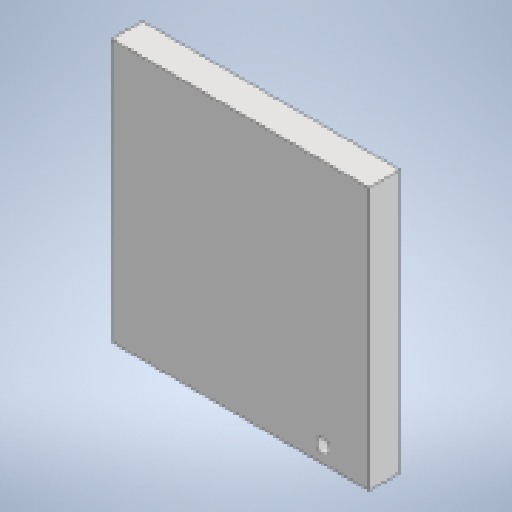
# Autodesk Inventor part: head_side
Saved by Autodesk Inventor 2024 (Build 280153000, 153)
## iProperties
Created: 2024-09-18
Part Number: head_side
Material: 일반
Document SubType Name: Modeling
Designer: Eungang
Density: 1 g/cm^3
Appearance: 기본값
Author: Eungang
Autodesk Inventor part; units mm, degrees
ref_plane "YZ Plane" through (0, 0, 0) normal (1, 0, 0) x (0, 1, 0)
ref_plane "XZ Plane" through (0, 0, 0) normal (0, 1, 0) x (-1, 0, 0)
ref_plane "XY Plane" through (0, 0, 0) normal (0, 0, 1) x (1, 0, 0)
sketch "스케치1" plane through (0, 0, 0) normal (0, 0, 1) x (1, 0, 0)
  line L0 (0, 0) -> (50, 0) projected
  line L1 (50, 0) -> (50, 25) projected
  line L2 (0, 25) -> (50, 25) projected
  line L3 (0, 0) -> (0, 25) projected
  line L4 (8.4, 0) -> (0, 0) projected
  line L5 (0, 0) -> (0, -16) projected
  line L6 (50, -16) -> (0, -16) projected
  line L7 (50, 0) -> (50, -16) projected
  line L8 (50, 0) -> (41.6, 0) projected
  line L9 (41.6, 0) -> (41.6, -10) projected
  line L10 (41.6, -10) -> (8.4, -10) projected
  line L11 (8.4, 0) -> (8.4, -10) projected
  line L12 (0, 25) -> (50, 25)
  line L13 (50, 25) -> (50, 35)
  line L14 (50, 35) -> (0, 35)
  line L15 (0, 35) -> (0, 25)
  line L16 (0, -16) -> (50, -16)
  line L17 (50, -16) -> (50, 35)
  line L18 (50, 35) -> (0, 35)
  line L19 (0, 35) -> (0, -16)
  dimension "d0" = 10
  constraints: 16 end point, 4 parallel, 2 horizontal, 2 perpendicular, 1 point on line
  measures "d0" distance of L13.end L12.end
extrude "돌출1" add sketch "스케치1" along normal blind 6
sketch "스케치2" plane through (0, 0, 6) normal (0, 0, 1) x (1, 0, 0)
  circle A0 centre (41, -13) radius 1.35 projected
  point P0 (0, 0)
extrude "돌출2" cut sketch "스케치2" against normal up to next
sketch "스케치3" plane through (0, 35, 0) normal (0, 1, 0) x (1, 0, 0)
  line L0 (50, 0) -> (0, 0) projected
  line L1 (28, -6) -> (50, -6) projected
  line L2 (39, -6) -> (25, 0)
  line L3 (39, -6) -> (22, -6)
  line L4 (22, -6) -> (22, 0)
  line L5 (22, 0) -> (39, 0)
  line L6 (39, 0) -> (39, -6)
  line L7 (39, 0) -> (28, 0)
  line L8 (28, 0) -> (28, -6)
  line L9 (28, -6) -> (39, -6)
  line L10 (39, -6) -> (39, 0)
  point P0 (22, -6)
  constraints: 18 end point, 4 parallel, 2 horizontal, 2 midpoint, 2 perpendicular, 2 point on line
extrude "돌출3" add sketch "스케치3" along normal blind 6 contours L8 L2 L0 | L2 L8 L3 L4 L0
sketch "스케치4" plane through (50, 35, 6) normal (0, 1, 0) x (1, 0, 0)
  circle A0 centre (-4.2, 79) radius 1.35 projected
  circle A1 centre (-4.2, 3) radius 1.35 projected
  circle A2 centre (-45.8, 79) radius 1.35 projected
  circle A3 centre (-45.8, 3) radius 1.35 projected
  circle A4 centre (-4.2, 71.8) radius 1.6 projected
  circle A5 centre (-45.8, 71.8) radius 1.6 projected
  circle A6 centre (-4.2, 10.2) radius 1.6 projected
  circle A7 centre (-45.8, 10.2) radius 1.6 projected
  line L0 (-50, 0) -> (-28, 0) projected
  line L1 (-28, 0) -> (-28, 6) projected
  line L2 (-28, 6) -> (-22, 6) projected
  line L3 (-22, 6) -> (-22, 0) projected
  line L4 (-22, 0) -> (0, 0) projected
  line L5 (0, 0) -> (0, 82) projected
  line L6 (0, 82) -> (-50, 82) projected
  line L7 (-50, 82) -> (-50, 0) projected
  point P0 (-50, 6)
extrude "돌출4" cut sketch "스케치4" against normal blind 6 contours A1 | A3
sketch "스케치6" plane through (0, 0, 6) normal (0, 0, 1) x (1, 0, 0)
  line L0 (47.05, 26.225) -> (47.05, 40.9)
  line L1 (47.05, 31.225) -> (47.05, 40.9)
  line L2 (47.05, 26.225) -> (49.65, 26.225)
  line L3 (50, -16) -> (50, 35) projected
  line L4 (47.05, 26.225) -> (44.45, 26.225)
  line L5 (44.45, 26.225) -> (44.45, 28.425)
  line L6 (44.45, 28.425) -> (49.65, 28.425)
  line L7 (49.65, 28.425) -> (49.65, 26.225)
  line L8 (28, 41) -> (22, 41) projected
  line L9 (25, 41) -> (25, 38)
  line L10 (2.95, 26.225) -> (0.35, 26.225)
  line L11 (2.95, 26.225) -> (5.55, 26.225)
  line L12 (5.55, 26.225) -> (5.55, 28.425)
  line L13 (5.55, 28.425) -> (0.35, 28.425)
  line L14 (0.35, 28.425) -> (0.35, 26.225)
  line L15 (0, 35) -> (0, -16) projected
  line L16 (0.35, 26.225) -> (0, 26.225)
  line L17 (0, 26.225) -> (0, 28.425)
  line L18 (0, 28.425) -> (0.35, 28.425)
  line L19 (0.35, 28.425) -> (0.35, 26.225)
  line L20 (49.65, 28.425) -> (50, 28.425)
  line L21 (50, 28.425) -> (50, 26.225)
  line L22 (50, 26.225) -> (49.65, 26.225)
  line L23 (49.65, 26.225) -> (49.65, 28.425)
  line L24 (0, 9.5) -> (2.95, 9.5)
  line L25 (47.05, -7.225) -> (49.65, -7.225)
  line L26 (47.05, -7.225) -> (44.45, -7.225)
  line L27 (44.45, -7.225) -> (44.45, -9.425)
  line L28 (44.45, -9.425) -> (49.65, -9.425)
  line L29 (49.65, -9.425) -> (49.65, -7.225)
  line L30 (2.95, -7.225) -> (0.35, -7.225)
  line L31 (2.95, -7.225) -> (5.55, -7.225)
  line L32 (5.55, -7.225) -> (5.55, -9.425)
  line L33 (5.55, -9.425) -> (0.35, -9.425)
  line L34 (0.35, -9.425) -> (0.35, -7.225)
  line L35 (0.35, -7.225) -> (0, -7.225)
  line L36 (0, -7.225) -> (0, -9.425)
  line L37 (0, -9.425) -> (0.35, -9.425)
  line L38 (0.35, -9.425) -> (0.35, -7.225)
  line L39 (49.65, -9.425) -> (50, -9.425)
  line L40 (50, -9.425) -> (50, -7.225)
  line L41 (50, -7.225) -> (49.65, -7.225)
  line L42 (49.65, -7.225) -> (49.65, -9.425)
  point P0 (0, 0)
  point P1 (47.05, -12.225)
  point P2 (0, -7.225)
  point P3 (0, 26.225)
  dimension "d11" = 2.6
  dimension "d12" = 2.6
  dimension "d13" = 2.2
  constraints: 80 end point, 22 symmetric about line, 5 horizontal, 5 perpendicular, 4 parallel, 4 point on line, 3 vertical, 2 midpoint, 3 other
  measures "d11" distance of L0.start L2.end
  measures "d12" distance of L0.start L4.end
  measures "d13" distance of L4.end L5.end
extrude "돌출6" cut sketch "스케치6" against normal up to next
sketch "스케치7" plane through (0, -16, 0) normal (0, -1, 0) x (1, 0, 0)
  line L0 (42.25, -2.775) -> (42.25, 11.9)
  line L1 (39.75, -2.775) -> (39.75, 11.9)
  line L2 (42.25, -2.775) -> (39.75, -2.775)
  line L3 (41, -2.775) -> (41, 6)
  line L4 (41, 0) -> (41, 6)
  line L5 (41, 3) -> (43.6, 3)
  line L6 (41, 3) -> (38.4, 3)
  line L7 (43.6, 3) -> (38.4, 3)
  line L8 (38.4, 3) -> (38.4, 1.9)
  line L9 (38.4, 1.9) -> (43.6, 1.9)
  line L10 (43.6, 1.9) -> (43.6, 3)
  line L11 (38.4, 3) -> (38.4, 4.1)
  line L12 (38.4, 4.1) -> (43.6, 4.1)
  line L13 (43.6, 4.1) -> (43.6, 3)
  point P0 (0, 0)
  dimension "d16" = 2.6
  dimension "d17" = 2.6
  dimension "d18" = 1.1
  constraints: 28 end point, 3 perpendicular, 3 vertical, 2 horizontal, 2 midpoint, 2 parallel, 2 symmetric about line, 1 collinear, 1 point on line, 4 other
  measures "d16" distance of L5.start L5.end
  measures "d17" distance of L5.start L6.end
  measures "d18" distance of L8.end L7.end
extrude "돌출7" cut sketch "스케치7" against normal blind 6 contours L9 L3 L5 L0 | L0 L5 L10 L9 | L5 L3 L12 L0 | L0 L12 L13 L5 | L9 L1 L6 L3 | L6 L1 L12 L3 | L9 L8 L6 L1 | L6 L11 L12 L1
